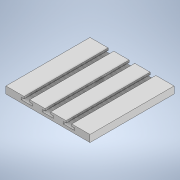
# Autodesk Inventor part: base plate
Saved by Autodesk Inventor 2022 (Build 260153000, 153)
## iProperties
Created: 2021-06-20
Part Number: base plate
Material: Generic
Document SubType Name: Modeling
Designer: WASHINGTON
Density: 1 g/cm^3
Appearance: Default
Author: WASHINGTON
Autodesk Inventor part; units mm, degrees
ref_plane "YZ Plane" through (0, 0, 0) normal (1, 0, 0) x (0, 1, 0)
ref_plane "XZ Plane" through (0, 0, 0) normal (0, 1, 0) x (-1, 0, 0)
ref_plane "XY Plane" through (0, 0, 0) normal (0, 0, 1) x (1, 0, 0)
sketch "Sketch1" plane through (0, 0, 0) normal (0, 0, 1) x (1, 0, 0)
  line L0 (-300, 0) -> (300, 0)
  line L1 (300, 0) -> (300, 50)
  line L2 (-300, 50) -> (-300, 0)
  line L3 (-20, 50) -> (-20, 35)
  line L4 (-20, 35) -> (-40, 35)
  line L5 (-40, 35) -> (-40, 20)
  line L6 (-40, 20) -> (40, 20)
  line L7 (40, 20) -> (40, 35)
  line L8 (40, 35) -> (20, 35)
  line L9 (20, 35) -> (20, 50)
  line L10 (-75, 159.793) -> (-75, -97.8722) construction
  line L11 (75, 159.793) -> (75, -92.8199) construction
  line L12 (-130, 50) -> (-130, 35)
  line L13 (-130, 35) -> (-110, 35)
  line L14 (-110, 35) -> (-110, 20)
  line L15 (-110, 20) -> (-190, 20)
  line L16 (-190, 20) -> (-190, 35)
  line L17 (-190, 35) -> (-170, 35)
  line L18 (-170, 35) -> (-170, 50)
  line L19 (170, 50) -> (170, 35)
  line L20 (170, 35) -> (190, 35)
  line L21 (190, 35) -> (190, 20)
  line L22 (190, 20) -> (110, 20)
  line L23 (110, 20) -> (110, 35)
  line L24 (110, 35) -> (130, 35)
  line L25 (130, 35) -> (130, 50)
  line L26 (-20, 50) -> (-130, 50)
  line L27 (-170, 50) -> (-300, 50)
  line L28 (300, 50) -> (170, 50)
  line L29 (130, 50) -> (20, 50)
  point P0 (0, 0)
  dimension "d0" = 300
  dimension "d1" = 600
  dimension "d2" = 50
  dimension "d3" = 50
  dimension "d4" = 20
  dimension "d5" = 20
  dimension "d6" = 20
  dimension "d7" = 20
  dimension "d8" = 30
  dimension "d9" = 15
  dimension "d10" = 15
  dimension "d12" = 75
  dimension "d13" = 75
  dimension "d14" = 15
  dimension "d15" = 109.793
  dimension "d16" = 142.8199
  dimension "d17" = 109.793
  dimension "d18" = 147.8722
  constraints: 60 end point, 16 symmetric about line, 9 perpendicular, 5 parallel, 4 vertical, 1 horizontal
  measures "d0" distance of point (0, 0) L0.start
  measures "d1" distance of L0.start L0.end
  measures "d2" distance of L2.start L0.start
  measures "d3" vertical distance of point (0, 0) L2.start
  measures "d4" horizontal distance of point (0, 0) L3.start
  measures "d5" horizontal distance of point (0, 0) L9.end
  measures "d6" distance of L3.end L4.end
  measures "d7" distance of L7.end L8.end
  measures "d8" vertical distance of L3.start L5.end
  measures "d9" distance of L4.end L5.end
  measures "d10" distance of L8.end L9.end
  measures "d12" distance from line of point (0, 0) L11
  measures "d13" distance from line of point (0, 0) L10
  measures "d14" distance between parallel lines of L24 L28
  measures "d15" distance from line of L11.start L28
  measures "d16" distance from line of L11.end L28
  measures "d17" distance from line of L10.start L28
  measures "d18" distance from line of L10.end L28
extrude "Extrusion1" add sketch "Sketch1" along normal mid plane 600
body "Solid1"
